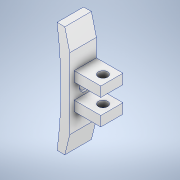
# Autodesk Inventor part: Schaufel_newtest
Saved by Autodesk Inventor 2021 (Build 250183000, 183)
## iProperties
Created: 2022-04-07
Part Number: Schaufel_newtest
Material: Aluminium 6061
Document SubType Name: Modeling
Designer: Timo
Density: 2.7 g/cm^3
Appearance: Aluminium - flach
Mass: 7.65892 g
Surface Area: 21.5996 cm^2
Volume: 2.83664 cm^3
Author: Timo
Autodesk Inventor part; units mm, degrees
ref_plane "YZ Plane" through (0, 0, 0) normal (1, 0, 0) x (0, 1, 0)
ref_plane "XZ Plane" through (0, 0, 0) normal (0, 1, 0) x (-1, 0, 0)
ref_plane "XY Plane" through (0, 0, 0) normal (0, 0, 1) x (1, 0, 0)
sketch "Skizze1" plane through (0, 0, 0) normal (0, 0, 1) x (1, 0, 0)
  line L0 (-7, 25) -> (0, 25)
  line L1 (0, 25) -> (0, -25)
  line L2 (0, -25) -> (-7, -25)
  line L3 (-7, -25) -> (-7, 25)
  point P0 (0, 0)
  point P1 (0, 0)
  dimension "d0" = 7
  dimension "d1" = 50
  constraints: 8 end point, 2 coincident, 2 parallel, 1 horizontal, 1 midpoint, 1 perpendicular
  measures "d0" distance between parallel lines of L3 L1
  measures "d1" distance of L0.end L1.end
extrude "Extrusion1" add sketch "Skizze1" along normal blind 12
sketch "Skizze2" plane through (0, -25, 0) normal (1, 0, 0) x (0, 0, -1)
  line L0 (-10, 33) -> (0, 33)
  line L1 (0, 33) -> (0, 17)
  line L2 (0, 17) -> (-10, 17)
  line L3 (-10, 17) -> (-10, 33)
  line L4 (0, 0) -> (0, 50) projected
  line L5 (-12, 0) -> (-12, 50) projected
  point P0 (0, 25)
  point P1 (0, 25)
  point P2 (0, 25)
  dimension "d4" = 0
  dimension "d6" = 16
  dimension "d48" = 10
  constraints: 8 end point, 2 midpoint, 2 parallel, 1 coincident, 1 horizontal, 1 perpendicular
  measures "d4" distance between parallel lines of L4 L1
  measures "d6" distance between parallel lines of L0 L2
  measures "d48" distance between parallel lines of L3 L1
extrude "Extrusion2" add sketch "Skizze2" along normal blind 12
sketch "Skizze5" plane through (0, 0, 12) normal (0, 0, 1) x (1, 0, 0)
  line L0 (12, -3.525) -> (0, -3.525)
  line L1 (0, -3.525) -> (0, 3.525)
  line L2 (0, 3.525) -> (12, 3.525)
  line L3 (12, 3.525) -> (12, -3.525)
  line L4 (12, -3.525) -> (0, 3.525) construction
  line L5 (0, -3.525) -> (12, 3.525) construction
  line L6 (12, 8) -> (12, -8) projected
  point P0 (0, 0)
  point P1 (6, 0)
  point P2 (6, 0)
  point P3 (0, 0)
  point P4 (6, 0)
  dimension "d27" = 7.05
  constraints: 12 end point, 5 midpoint, 2 horizontal alignment, 2 parallel, 1 horizontal, 1 perpendicular, 1 point on line, 1 vertical alignment
  measures "d27" distance of L0.end L1.end
extrude "Extrusion3" cut sketch "Skizze5" against normal through all
sketch "Skizze6" plane through (0, 8, 12) normal (0, 1, 0) x (1, 0, 0)
  line L0 (0, 2) -> (0, 12) construction
  line L1 (0, 2) -> (12, 2) construction
  line L2 (12, 12) -> (12, 2) construction
  line L3 (0, 12) -> (12, 12) construction
  point P0 (0, 12)
  point P1 (8, 7)
  point P2 (12, 7)
  point P3 (6, 2)
  dimension "d38" = 8
  dimension "d47" = 5
  constraints: 2 midpoint
  measures "d38" distance from line of L0 point (8, 7)
  measures "d47" distance from line of L1 point (8, 7)
hole "Bohrung3" at (8, 8, 5) direction (0, -1, 0) diameter 4.2 end through all
sketch "Skizze7" plane through (0, -3.525, 12) normal (1, 0, 0) x (0, 0, -1)
  line L0 (12, 7.05) -> (12, 0) construction
  line L1 (2, 7.05) -> (12, 7.05) construction
  line L2 (0, -21.475) -> (0, 28.525) construction
  line L3 (2, 0) -> (12, 0) construction
  line L4 (12, 0) -> (2, 0) projected
  line L5 (12, -21.475) -> (0, -21.475) projected
  line L6 (12, -21.475) -> (12, -4.475) projected
  line L7 (12, -4.475) -> (2, -4.475) projected
  line L8 (2, -4.475) -> (2, 0) projected
  line L9 (2, 7.05) -> (2, 11.525) projected
  line L10 (2, 11.525) -> (12, 11.525) projected
  line L11 (12, 11.525) -> (12, 28.525) projected
  line L12 (12, 28.525) -> (0, 28.525) projected
  line L13 (2, 7.05) -> (12, 7.05) projected
  point P0 (12, 3.525)
  point P1 (0, 0)
  point P2 (7, 3.525)
  point P3 (7, 0)
  point P4 (0, 3.525)
  point P5 (7, 7.05)
  constraints: 3 midpoint, 1 horizontal alignment, 1 vertical alignment
hole "Bohrung4" at (0, 0, 5) direction (-1, 0, 0) diameter 4.2 end through all
sketch "Skizze9" plane through (0, 0, 12) normal (0, 0, 1) x (1, 0, 0)
  line L0 (-7, -25) -> (0, -25) projected
  line L1 (0, -25) -> (0, 25) projected
  line L2 (0, 25) -> (-7, 25) projected
  line L3 (-7, 25) -> (-7, -25) projected
  arc A0 (-5.7446, -25) -> (-5.7446, 25) centre (-184, 0) ccw
  line L4 (0, -8) -> (12, -8) projected
  line L5 (-4, 0) -> (0, 0) construction
  line L6 (-2.2446, 25) -> (0, 16)
  line L7 (0, 8) -> (12, 8) projected
  line L8 (0, -16) -> (-2.2446, -25)
  point P0 (0, 0)
  dimension "d55" = 4
  dimension "d56" = 180
  dimension "d57" = 8
  dimension "d58" = 3.5
  dimension "d59" = 8
  dimension "d60" = 3.5
  constraints: 6 end point, 6 point on line, 3 point on circle, 1 centre point, 1 horizontal alignment, 1 midpoint, 1 perpendicular, 1 vertical alignment
  measures "d55" distance of L5.start L5.end
  measures "d56" radius of A0
  measures "d57" distance from line of L7 L6.end
  measures "d58" distance of L6.start A0.end
  measures "d59" distance of L4.start L8.start
  measures "d60" distance of L8.end A0.start
extrude "Extrusion4" cut sketch "Skizze9" against normal through all contours L3 L2 A0 L0 | L8 L1 L0 | L2 L1 L6
chamfer "Fase1" distance 0.5 angle 45 1 edges at (0, 0, 7.1)
